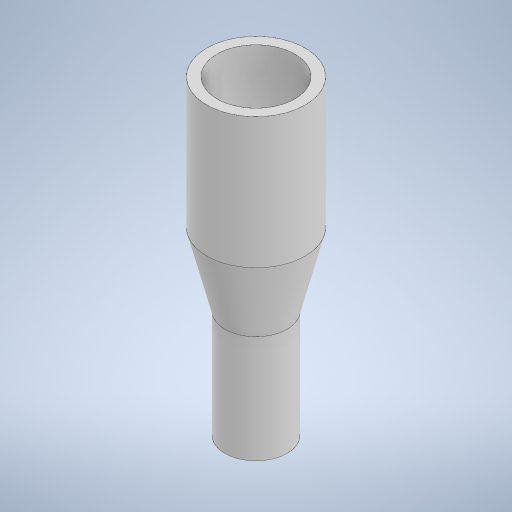
# Autodesk Inventor part: piston
Saved by Autodesk Inventor 2024.2 (Build 282272000, 272)
## iProperties
Created: 2024-05-29
Part Number: piston
Material: Generic
Document SubType Name: Modeling
Designer: user
Density: 1 g/cm^3
Appearance: Default
Author: user
Autodesk Inventor part; units mm, degrees
ref_plane "YZ Plane" through (0, 0, 0) normal (1, 0, 0) x (0, 1, 0)
ref_plane "XZ Plane" through (0, 0, 0) normal (0, 1, 0) x (-1, 0, 0)
ref_plane "XY Plane" through (0, 0, 0) normal (0, 0, 1) x (1, 0, 0)
sketch "Sketch1" plane through (0, 0, 0) normal (0, 0, 1) x (1, 0, 0)
  line L0 (0, 0) -> (0, 120)
  line L1 (0, 120) -> (19, 120)
  line L2 (19, 120) -> (19, 69.5)
  line L3 (0, 0) -> (12, 0)
  line L4 (12, 0) -> (12, 41.5)
  line L5 (0, -24) -> (0, 144) projected
  line L6 (12, 41.5) -> (12, 50)
  line L7 (12, 41.5) -> (19, 69.5)
  line L8 (12, 50) -> (14.125, 50)
  dimension "d0" = 120
  dimension "d1" = 19
  dimension "d2" = 50.5
  dimension "d3" = 12
  dimension "d4" = 41.5
  dimension "d7" = 8.5
  constraints: 16 end point, 3 vertical, 2 horizontal, 2 perpendicular, 1 point on line
  measures "d0" distance of L0.start L0.end
  measures "d1" distance of L0.end L1.end
  measures "d2" distance of L1.end L2.end
  measures "d3" distance of L0.start L3.end
  measures "d4" distance of L3.end L4.end
  measures "d7" distance of L4.end L6.end
revolve "Revolution1" add sketch "Sketch1" angle 360 about axis through (0, -10, 0) along (0, 1, 0) contours L0 L1 L2 L7 L8 L6 L4 L3
shell "Shell1" thickness 4 removed faces 2 at (4.7406, 120, 4.1998) at (0.4821, 0, -1.3341)
sketch "Sketch2" plane through (0, 0, 0) normal (0, 0, 1) x (1, 0, 0)
  line L0 (14.125, 50) -> (-14.125, 50) projected
  line L1 (-12, 0) -> (-12, 50) projected
  line L2 (-14.125, 50) -> (-12, 41.5)
  line L3 (-14.125, 50) -> (-19, 69.5) projected
  line L4 (-14.125, 50) -> (-12, 50)
  line L5 (-12, 50) -> (-12, 41.5)
  line L6 (0, -24) -> (0, 144) projected
  point P0 (0, 0)
  constraints: 6 end point, 2 collinear, 1 perpendicular, 1 point on line
revolve "Revolution2" add sketch "Sketch2" angle 360 about axis through (0, -10, 0) along (0, 1, 0)
body "Solid1"
